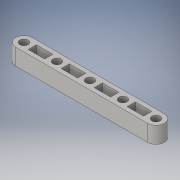
# Autodesk Inventor part: 4M Module
Saved by Autodesk Inventor 2016 SP1 (Build 200210100, 210)
## iProperties
Created: 2016-02-02
Part Number: 4M Module
Material: Wood (Oak)
Document SubType Name: Modeling
Designer: jleonard
Density: 0.76 g/cm^3
Appearance: White Oak - Natural Medium Gloss
Author: jleonard
Autodesk Inventor part; units mm, degrees
ref_plane "YZ Plane" through (0, 0, 0) normal (1, 0, 0) x (0, 1, 0)
ref_plane "XZ Plane" through (0, 0, 0) normal (0, 1, 0) x (-1, 0, 0)
ref_plane "XY Plane" through (0, 0, 0) normal (0, 0, 1) x (1, 0, 0)
sketch "Sketch1" plane through (0, 0, 0) normal (0, 1, 0) x (-1, 0, 0)
  line L0 (50.8, 6.35) -> (-50.8, 6.35)
  line L1 (-50.8, -6.35) -> (50.8, -6.35)
  arc A0 (50.8, -6.35) -> (50.8, 6.35) centre (50.8, 0) ccw
  arc A1 (-50.8, 6.35) -> (-50.8, -6.35) centre (-50.8, 0) ccw
  line L2 (80.01, 0) -> (-80.01, 0) projected
  line L3 (0, -8.89) -> (0, 8.89) projected
  point P0 (0, 0)
  dimension "d2" = 101.6
  dimension "d3" = 6.35
  dimension "d4" = 6.35
  dimension "d5" = 50.8
  dimension "d6" = 0
  dimension "d7" = 12.7
  dimension "d8" = 101.6
  dimension "d9" = 6.35
  constraints: 4 end point, 4 point on circle, 2 centre point, 1 horizontal, 1 parallel
  measures "d2" distance of A1.centre A0.centre
  measures "d3" radius of A1
  measures "d4" radius of A0
  measures "d5" distance from line of A1.centre L3
  measures "d6" distance from line of L2 A1.centre
  measures "d7" distance between parallel lines of L1 L0
  measures "d8" distance of L0.start L0.end
  measures "d9" distance from line of L1 A0.centre
extrude "Extrusion1" add sketch "Sketch1" along normal blind 12.7
sketch "Sketch2" plane through (0, 12.7, 0) normal (0, 1, 0) x (1, 0, 0)
  circle A0 centre (-50.8, 0) radius 3.175
  line L0 (-80.01, 0) -> (80.01, 0) projected
  line L1 (0, 8.89) -> (0, -8.89) projected
  circle A1 centre (-25.4, 0) radius 3.175
  circle A2 centre (0, 0) radius 3.175
  circle A3 centre (25.4, 0) radius 3.175
  circle A4 centre (50.8, 0) radius 3.175
  dimension "d12" = 6.35
  dimension "d13" = 50.8
  dimension "d14" = 0
  dimension "d17" = 25.4
  constraints: 5 centre point, 1 horizontal, 8 other
  measures "d12" diameter of A0
  measures "d13" distance from line of L1 A0.centre
  measures "d14" distance from line of L0 A0.centre
  measures "d17" distance of A0.centre A1.centre
extrude "Extrusion2" cut sketch "Sketch2" against normal through all
sketch "Sketch3" plane through (0, 12.7, 0) normal (0, 1, 0) x (1, 0, 0)
  line L0 (-44.45, -3.175) -> (-31.75, -3.175)
  line L1 (-31.75, -3.175) -> (-31.75, 3.175)
  line L2 (-31.75, 3.175) -> (-44.45, 3.175)
  line L3 (-44.45, 3.175) -> (-44.45, -3.175)
  line L4 (-84.8983, 0) -> (80.8247, 0) projected
  line L5 (0, 12.3762) -> (0, -29.8073) projected
  line L6 (-6.35, 3.175) -> (-19.05, 3.175)
  line L7 (-6.35, -3.175) -> (-6.35, 3.175)
  line L8 (-19.05, 3.175) -> (-19.05, -3.175)
  line L9 (-19.05, -3.175) -> (-6.35, -3.175)
  line L10 (19.05, 3.175) -> (6.35, 3.175)
  line L11 (19.05, -3.175) -> (19.05, 3.175)
  line L12 (6.35, 3.175) -> (6.35, -3.175)
  line L13 (6.35, -3.175) -> (19.05, -3.175)
  line L14 (44.45, 3.175) -> (31.75, 3.175)
  line L15 (44.45, -3.175) -> (44.45, 3.175)
  line L16 (31.75, 3.175) -> (31.75, -3.175)
  line L17 (31.75, -3.175) -> (44.45, -3.175)
  point P0 (0, 0)
  dimension "d24" = 12.7
  dimension "d25" = 6.35
  dimension "d26" = 31.75
  dimension "d27" = 3.175
  dimension "d30" = 25.4
  constraints: 32 end point, 2 horizontal, 2 parallel, 1 perpendicular, 24 other
  measures "d24" distance of L0.start L0.end
  measures "d25" distance of L0.end L1.end
  measures "d26" distance between parallel lines of L5 L1
  measures "d27" distance between parallel lines of L4 L0
  measures "d30" distance of L1.end L6.start
extrude "Extrusion3" cut sketch "Sketch3" against normal through all
body "Solid1"
